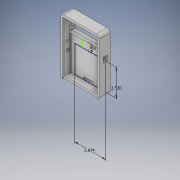
# Autodesk Inventor part: Capstone Calculator
Saved by Autodesk Inventor 2018 (Build 220112000, 112)
## iProperties
Created: 2019-09-20
Part Number: Capstone Calculator
Material: Generic
Document SubType Name: Modeling
Designer: Hyperspin
Density: 1 g/cm^3
Appearance: Default
Author: Hyperspin
Autodesk Inventor part; units mm, degrees
ref_plane "YZ Plane" through (0, 0, 0) normal (1, 0, 0) x (0, 1, 0)
ref_plane "XZ Plane" through (0, 0, 0) normal (0, 1, 0) x (-1, 0, 0)
ref_plane "XY Plane" through (0, 0, 0) normal (0, 0, 1) x (1, 0, 0)
sketch "Sketch1" plane through (0, 0, 0) normal (0, 0, 1) x (1, 0, 0)
  line L0 (0, 0) -> (71, 0)
  line L1 (71, 0) -> (71, 78)
  line L2 (71, 78) -> (0, 78)
  line L3 (0, 78) -> (0, 0)
  line L4 (-4.8, 123.3464) -> (76.2, 123.3464)
  line L5 (76.2, 123.3464) -> (76.2, 86.3464)
  line L6 (76.2, 86.3464) -> (-4.8, 86.3464)
  line L7 (-4.8, 86.3464) -> (-4.8, 123.3464)
  line L8 (-0.5, 90.3464) -> (71.5, 90.3464)
  line L9 (71.5, 90.3464) -> (71.5, 116.3464)
  line L10 (71.5, 116.3464) -> (-0.5, 116.3464)
  line L11 (-0.5, 116.3464) -> (-0.5, 90.3464)
  line L12 (24.5, 0) -> (46.5, 0)
  line L13 (24.5, 0) -> (46.5, 0)
  line L14 (46.5, 0) -> (46.5, 6)
  line L15 (46.5, 6) -> (24.5, 6)
  line L16 (24.5, 6) -> (24.5, 0)
  circle A0 centre (-2.1, 120.6464) radius 1.5
  circle A1 centre (73.5, 120.6464) radius 1.5
  circle A2 centre (-2.1, 89.0464) radius 1.5
  circle A3 centre (73.5, 89.0464) radius 1.5
  dimension "d0" = 71
  dimension "d1" = 78
  dimension "d2" = 37
  dimension "d3" = 81
  dimension "d4" = 72
  dimension "d5" = 26
  dimension "d6" = 4.7
  dimension "d7" = 7
  dimension "d9" = 0.5
  dimension "d14" = 6
  dimension "d15" = 3
  dimension "d16" = 2.7
  dimension "d17" = 2.7
  constraints: 34 end point, 8 parallel, 5 horizontal, 4 centre point, 4 perpendicular, 1 point on line
  measures "d0" distance of L1.end L2.end
  measures "d1" distance of L0.end L1.end
  measures "d2" distance of L4.end L5.end
  measures "d3" distance of L4.start L4.end
  measures "d4" distance of L9.end L10.end
  measures "d5" distance of L8.end L9.end
  measures "d6" distance between parallel lines of L5 L9
  measures "d7" distance between parallel lines of L4 L10
  measures "d9" distance between parallel lines of L3 L11
  measures "d14" distance of L13.end L14.end
  measures "d15" diameter of A0
  measures "d16" distance from line of L4 A0.centre
  measures "d17" distance from line of A0.centre L7
extrude "Extrusion1" add sketch "Sketch1" along normal blind 6.5 contours L3 L2 L1 L0 L14 L15 L16 | L4 L5 L6 L7
sketch "Sketch2" plane through (0, 0, 6.5) normal (0, 0, 1) x (1, 0, 0)
  line L0 (-2.8, 128.3464) -> (74.2, 128.3464)
  line L1 (81.2, 121.3464) -> (81.2, 2)
  line L2 (74.2, -5) -> (-2.8, -5)
  line L3 (-9.8, 2) -> (-9.8, 121.3464)
  line L4 (76.2, 86.3464) -> (76.2, 123.3464) projected
  line L5 (76.2, 123.3464) -> (-4.8, 123.3464) projected
  line L6 (-4.8, 123.3464) -> (-4.8, 86.3464) projected
  line L7 (46.5, 0) -> (71, 0) projected
  arc A0 (-2.8, 128.3464) -> (-9.8, 121.3464) centre (-2.8, 121.3464) ccw
  arc A1 (81.2, 121.3464) -> (74.2, 128.3464) centre (74.2, 121.3464) ccw
  arc A2 (-9.8, 2) -> (-2.8, -5) centre (-2.8, 2) ccw
  arc A3 (74.2, -5) -> (81.2, 2) centre (74.2, 2) ccw
  line L8 (76.2, 123.3464) -> (76.2, 86.3464) projected
  line L9 (-4.8, 123.3464) -> (76.2, 123.3464) projected
  line L10 (-4.8, 86.3464) -> (-4.8, 123.3464) projected
  line L11 (76.2, 86.3464) -> (-4.8, 86.3464) projected
  line L12 (46.5, 0) -> (71, 0) projected
  line L13 (71, 0) -> (0, 0)
  line L14 (0, 0) -> (0, 78)
  line L15 (0, 78) -> (71, 78)
  line L16 (71, 78) -> (71, 0)
  point P0 (0, 0)
  dimension "d20" = 5
  dimension "d21" = 5
  dimension "d22" = 5
  dimension "d23" = 5
  dimension "d24" = 7
  constraints: 16 end point, 8 point on circle, 8 tangent, 4 centre point, 4 parallel, 3 equal radius, 2 horizontal, 2 perpendicular
  measures "d20" distance between parallel lines of L1 L4
  measures "d21" distance between parallel lines of L0 L5
  measures "d22" distance between parallel lines of L3 L6
  measures "d23" distance between parallel lines of L2 L7
  measures "d24" radius of A0
extrude "Extrusion2" add sketch "Sketch2" against normal blind 8.5
sketch "Sketch3" plane through (0, 0, 0) normal (0, 0, -1) x (-1, 0, 0)
  line L0 (-76.2, 86.3464) -> (-76.2, 123.3464) projected
  line L1 (-76.2, 86.3464) -> (4.8, 86.3464) projected
  line L2 (-76.2, 123.3464) -> (4.8, 123.3464)
  line L3 (4.8, 123.3464) -> (4.8, 86.3464)
  line L4 (4.8, 86.3464) -> (-76.2, 86.3464)
  line L5 (-76.2, 86.3464) -> (-76.2, 123.3464)
  line L6 (-71.5, 116.3464) -> (-71.5, 90.3464) projected
  line L7 (0.5, 116.3464) -> (0.5, 90.3464) projected
  line L8 (-71.5, 116.3464) -> (0.5, 116.3464)
  line L9 (0.5, 116.3464) -> (0.5, 90.3464)
  line L10 (0.5, 90.3464) -> (-71.5, 90.3464)
  line L11 (-71.5, 90.3464) -> (-71.5, 116.3464)
  point P0 (0, 0)
  constraints: 16 end point, 4 parallel, 2 horizontal, 2 perpendicular
extrude "Extrusion3" add sketch "Sketch3" along normal up to surface (2 mm away)
sketch "Sketch4" plane through (0, 0, 6.5) normal (0, 0, 1) x (1, 0, 0)
  line L0 (71.5, 116.3464) -> (71.5, 90.3464) projected
  line L1 (-0.5, 116.3464) -> (71.5, 116.3464) projected
  line L2 (71.5, 90.3464) -> (-0.5, 90.3464) projected
  line L3 (0.5, 116.3464) -> (41.5, 116.3464)
  line L4 (-0.5, 90.3464) -> (-0.5, 116.3464) projected
  line L5 (-2.8, 128.3464) -> (74.2, 128.3464) projected
  line L6 (-0.5, 116.3464) -> (-0.5, 90.3464)
  line L7 (-0.5, 96.0971) -> (-5.5585, 96.0971)
  line L8 (-5.5585, 96.0971) -> (-5.5585, 110.5971)
  line L9 (-5.5585, 110.5971) -> (-0.5, 110.5971)
  line L10 (71.5, 116.3464) -> (-0.5, 116.3464)
  line L11 (28.5, 116.3464) -> (28.5, 123.3464)
  line L12 (28.5, 123.3464) -> (70.5, 123.3464)
  line L13 (70.5, 123.3464) -> (70.5, 116.3464)
  line L14 (28.5, 116.3464) -> (70.5, 116.3464)
  line L15 (-0.5, 96.0971) -> (-0.5, 110.5971)
  point P0 (0, 0)
  point P1 (71.5, 96.0971)
  dimension "d37" = 1
  dimension "d38" = 42
  constraints: 22 end point, 4 point on line, 1 collinear, 1 horizontal, 1 vertical
  measures "d37" distance between parallel lines of L13 L0
  measures "d38" distance of L12.start L12.end
extrude "Extrusion4" cut sketch "Sketch4" against normal blind 4
sketch "Sketch5" plane through (0, 0, 6.5) normal (0, 0, 1) x (1, 0, 0)
  line L0 (-4.8, 83.3464) -> (76.2, 83.3464)
  line L1 (76.2, 83.3464) -> (76.2, 0)
  line L2 (76.2, 0) -> (-4.8, 0)
  line L3 (-4.8, 0) -> (-4.8, 83.3464)
  line L4 (-9.8, 2) -> (-9.8, 121.3464) projected
  line L5 (81.2, 121.3464) -> (81.2, 2) projected
  line L6 (71.5, 90.3464) -> (-0.5, 90.3464) projected
  line L7 (46.5, 0) -> (24.5, 0) projected
  point P0 (0, 0)
  dimension "d41" = 5
  dimension "d42" = 5
  dimension "d43" = 7
  dimension "d44" = 0
  constraints: 8 end point, 2 parallel, 1 horizontal, 1 perpendicular
  measures "d41" distance between parallel lines of L3 L4
  measures "d42" distance between parallel lines of L5 L1
  measures "d43" distance between parallel lines of L6 L0
  measures "d44" distance between parallel lines of L7 L2
extrude "Extrusion5" cut sketch "Sketch5" against normal blind 3
sketch "Sketch7" plane through (0, 0, 6.5) normal (0, 0, 1) x (1, 0, 0)
  line L0 (28.5, 116.3464) -> (28.5, 123.3464) projected
  line L1 (28.5, 123.3464) -> (70.5, 123.3464) projected
  line L2 (70.5, 123.3464) -> (70.5, 116.3464) projected
  line L3 (70.5, 116.3464) -> (71.5, 116.3464) projected
  line L4 (71.5, 116.3464) -> (71.5, 90.3464) projected
  line L5 (71.5, 90.3464) -> (-0.5, 90.3464) projected
  line L6 (-0.5, 90.3464) -> (-0.5, 96.0971) projected
  line L7 (-0.5, 96.0971) -> (-5.5585, 96.0971) projected
  line L8 (-5.5585, 96.0971) -> (-5.5585, 110.5971) projected
  line L9 (-5.5585, 110.5971) -> (-0.5, 110.5971) projected
  line L10 (-0.5, 110.5971) -> (-0.5, 116.3464) projected
  line L11 (-0.5, 116.3464) -> (28.5, 116.3464) projected
  line L12 (76.2, 0) -> (-4.8, 0) projected
  line L13 (-4.8, 0) -> (-4.8, 83.3464) projected
  line L14 (-4.8, 83.3464) -> (76.2, 83.3464) projected
  line L15 (76.2, 83.3464) -> (76.2, 0) projected
  line L16 (-2.8, 128.3464) -> (74.2, 128.3464) projected
  arc A0 (-2.8, 128.3464) -> (-9.8, 121.3464) centre (-2.8, 121.3464) ccw projected
  line L17 (-9.8, 2) -> (-9.8, 121.3464) projected
  arc A1 (-9.8, 2) -> (-2.8, -5) centre (-2.8, 2) ccw projected
  line L18 (74.2, -5) -> (-2.8, -5) projected
  arc A2 (74.2, -5) -> (81.2, 2) centre (74.2, 2) ccw projected
  line L19 (81.2, 121.3464) -> (81.2, 2) projected
  arc A3 (81.2, 121.3464) -> (74.2, 128.3464) centre (74.2, 121.3464) ccw projected
  circle A4 centre (73.5, 89.0464) radius 1.5 projected
  circle A5 centre (-2.1, 89.0464) radius 1.5 projected
  circle A6 centre (73.5, 120.6464) radius 1.5 projected
  circle A7 centre (-2.1, 120.6464) radius 1.5 projected
  line L20 (-4.8, 83.3464) -> (76.2, 83.3464)
  line L21 (76.962, 83.3464) -> (76.962, 123.3464)
  line L22 (76.962, 123.3464) -> (-5.5585, 123.3464)
  line L23 (-5.5585, 123.3464) -> (-5.5585, 83.3464)
  line L24 (76.962, 83.3464) -> (76.962, 0)
  line L25 (76.2, 83.3464) -> (76.2, 0) projected
  line L26 (76.962, 0) -> (76.2, 0)
  line L27 (-5.5585, 83.3464) -> (-5.5585, 0)
  line L28 (-5.5585, 0) -> (-4.8, 0)
  point P0 (0, 0)
  dimension "d51" = 0.7585
  dimension "d52" = 0.762
  constraints: 16 end point, 4 perpendicular, 4 point on line, 2 parallel, 1 horizontal, 1 vertical
  measures "d51" distance between parallel lines of L23 L13
  measures "d52" distance between parallel lines of L21 L15
extrude "Extrusion7" add sketch "Sketch7" along normal blind 17 contours L16 A3 L19 A2 L18 A1 L17 A0
sketch "Sketch8" plane through (0, 0, 3.5) normal (0, 0, 1) x (1, 0, 0)
  line L0 (76.2, 83.3464) -> (76.2, 0) projected
  line L1 (76.2, 0) -> (3.2, 0)
  line L2 (3.2, 0) -> (3.2, 64)
  line L3 (3.2, 64) -> (76.2, 64)
  line L4 (76.2, 64) -> (76.2, 0)
  line L5 (33.6587, 64) -> (21.1159, 64)
  line L6 (21.1159, 64) -> (21.1159, 82)
  line L7 (21.1159, 82) -> (33.6587, 82)
  line L8 (33.6587, 82) -> (33.6587, 64)
  point P0 (0, 0)
  dimension "d55" = 73
  dimension "d56" = 64
  dimension "d57" = 18
  constraints: 16 end point, 4 parallel, 2 horizontal, 2 perpendicular, 1 point on line
  measures "d55" distance of L2.end L3.end
  measures "d56" distance between parallel lines of L1 L3
  measures "d57" distance of L7.end L5.start
sketch "Sketch9" plane through (-2.8, -5, -2) normal (0, -1, 0) x (1, 0, 0)
  line L0 (-2.7585, 8.5) -> (-2.7585, 25.5) projected
  line L1 (-2.7585, 21.5) -> (79.762, 21.5)
  line L2 (79.762, 23.5) -> (79.762, 25.5)
  line L3 (79.762, 25.5) -> (-2.7585, 25.5)
  line L4 (-2.7585, 25.5) -> (-2.7585, 23.5)
  line L5 (-2.7585, 21.5) -> (-4.7585, 21.5)
  line L6 (-4.7585, 21.5) -> (-4.7585, 23.5)
  line L7 (-4.7585, 23.5) -> (-2.7585, 23.5)
  line L8 (-2.7585, 23.5) -> (-2.7585, 21.5)
  line L9 (79.762, 25.5) -> (-2.7585, 25.5) projected
  line L10 (79.762, 21.5) -> (81.762, 21.5)
  line L11 (81.762, 21.5) -> (81.762, 23.5)
  line L12 (81.762, 23.5) -> (79.762, 23.5)
  point P0 (2.8, 2)
  dimension "d58" = 4
  dimension "d59" = 2
  dimension "d60" = 2
  constraints: 22 end point, 4 parallel, 2 horizontal, 2 perpendicular, 1 point on line
  measures "d58" distance between parallel lines of L1 L3
  measures "d59" distance of L1.start L5.end
  measures "d60" distance of L5.end L6.end
extrude "Extrusion8" cut sketch "Sketch9" against normal up to surface (128.3464 mm away)
sketch "Sketch10" plane through (-9.8, 2, -2) normal (-1, 0, 0) x (0, 0, 1)
  line L0 (0, 0) -> (0, 119.3464) projected
  line L1 (25.5, -6.4335) -> (25.5, 121.3464) projected
  circle A0 centre (12.75, 77.5) radius 2.9
  line L2 (9.75, 63.5) -> (15.75, 63.5)
  line L3 (15.75, 63.5) -> (15.75, 69.5)
  line L4 (15.75, 69.5) -> (9.75, 69.5)
  line L5 (9.75, 69.5) -> (9.75, 63.5)
  point P0 (2, -2)
  dimension "d63" = 5.8
  dimension "d64" = 6
  dimension "d65" = 6
  dimension "d67" = 8
  dimension "d70" = 63.5
  constraints: 8 end point, 2 parallel, 1 centre point, 1 horizontal, 1 perpendicular
  measures "d63" diameter of A0
  measures "d64" distance of L3.end L4.end
  measures "d65" distance of L2.end L3.end
  measures "d67" distance from line of A0.centre L4
  measures "d70" distance from line of L2 L0.start
extrude "Extrusion9" cut sketch "Sketch10" against normal up to surface (4.2415 mm away)
sketch "Sketch11" plane through (76.962, 0, 6.5) normal (-1, 0, 0) x (0, 0, 1)
  point P0 (-6.5, 0)
sketch "Sketch12" plane through (76.962, 0, 6.5) normal (-1, 0, 0) x (0, 0, 1)
  line L0 (-6.1095, 84.0437) -> (-4.1453, 84.0437)
  line L1 (-4.1453, 84.0437) -> (-4.1453, 62.8671)
  line L2 (-4.1453, 62.8671) -> (-6.1095, 62.8671)
  line L3 (-6.1095, 62.8671) -> (-6.1095, 84.0437)
  line L4 (0, 0) -> (0, 123.3464) projected
  line L5 (0, 77.7054) -> (6, 77.7054)
  line L6 (6, 77.7054) -> (6, 69.2054)
  line L7 (6, 69.2054) -> (0, 69.2054)
  line L8 (0, 69.2054) -> (0, 77.7054)
  line L9 (-6.1095, 73.4554) -> (0, 73.4554)
  line L10 (6, 73.4554) -> (14.2516, 73.4554)
  point P0 (-6.5, 0)
  point P1 (13, 0)
  dimension "d71" = 6
  dimension "d72" = 8.5
  constraints: 20 end point, 4 horizontal, 4 parallel, 3 midpoint, 2 perpendicular, 1 point on line
  measures "d71" distance of L5.start L5.end
  measures "d72" distance of L5.end L6.end
extrude "Extrusion10" cut sketch "Sketch12" against normal up to surface (4.238 mm away) contours L4 L5 L6 L7
sketch "Sketch13" plane through (81.2, 2, -2) normal (1, 0, 0) x (0, 0, -1)
  line L0 (-8.5, 67.2054) -> (-14.5, 67.2054) projected
  line L1 (-14.5, 67.2054) -> (-14.5, 75.7054) projected
  line L2 (-14.5, 75.7054) -> (-8.5, 75.7054) projected
  line L3 (-8.5, 75.7054) -> (-8.5, 67.2054) projected
  line L4 (-16.4563, 77.6617) -> (-16.4563, 65.2491)
  line L5 (-16.4563, 65.2491) -> (-6.5437, 65.2491)
  line L6 (-6.5437, 65.2491) -> (-6.5437, 77.6617)
  line L7 (-6.5437, 77.6617) -> (-16.4563, 77.6617)
  point P0 (-2, -2)
  constraints: 8 end point, 3 other
extrude "Extrusion11" cut sketch "Sketch13" against normal blind 3
sketch "Sketch14" plane through (-5.5585, 0, 6.5) normal (1, 0, 0) x (0, 0, -1)
  line L0 (-1.25, 65.5) -> (-7.25, 65.5) projected
  line L1 (-7.5, 46.0518) -> (-1, 46.0518)
  line L2 (-1, 46.0518) -> (-1, 52.5518)
  line L3 (-1, 52.5518) -> (-7.5, 52.5518)
  line L4 (-7.5, 52.5518) -> (-7.5, 46.0518)
  line L5 (-4.25, 65.5) -> (-4.25, 49.9279)
  point P0 (6.5, 0)
  dimension "d79" = 6.5
  dimension "d80" = 6.5
  dimension "d81" = 3.25
  constraints: 10 end point, 2 parallel, 1 horizontal, 1 midpoint, 1 perpendicular, 1 vertical
  measures "d79" distance of L3.end L1.start
  measures "d80" distance of L1.start L1.end
  measures "d81" distance between parallel lines of L5 L4
extrude "Extrusion12" cut sketch "Sketch14" against normal blind 3
sketch "Sketch15" plane through (-9.8, 2, -2) normal (-1, 0, 0) x (0, 0, 1)
  line L0 (9.5, 50.5518) -> (9.5, 44.0518) projected
  line L1 (9.5, 44.0518) -> (16, 44.0518) projected
  line L2 (9.5, 50.5518) -> (9.5, 44.0518) projected
  line L3 (16, 50.5518) -> (9.5, 50.5518) projected
  line L4 (16, 44.0518) -> (16, 50.5518) projected
  circle A0 centre (12.75, 47.3018) radius 3.25
  line L5 (16, 44.0518) -> (16, 50.5518) projected
  point P0 (2, -2)
  constraints: 1 centre point, 1 tangent
extrude "Extrusion13" cut sketch "Sketch15" against normal up to surface (1.2415 mm away) contours A0
sketch "Sketch16" plane through (-2.8, -5, 19.5) normal (0, 0, 1) x (1, 0, 0)
  line L0 (-2.7585, 0.5665) -> (-2.7585, 128.3464) projected
  line L1 (-2.7585, 128.3464) -> (-2.7585, 5) projected
  arc A0 (-4.7585, 1.8662) -> (0, 0) centre (0, 7) ccw projected
  line L2 (77, 0) -> (0, 0) projected
  line L3 (-2.7585, 5) -> (79.762, 5) projected
  arc A1 (77, 0) -> (81.762, 1.8694) centre (77, 7) ccw projected
  line L4 (-4.7585, 128.3464) -> (-2.7585, 128.3464) projected
  arc A2 (-4.7585, 1.8662) -> (0, 0) centre (0, 7) ccw projected
  line L5 (77, 0) -> (0, 0) projected
  arc A3 (77, 0) -> (81.762, 1.8694) centre (77, 7) ccw projected
  line L6 (81.762, 1.8694) -> (81.762, 128.3464) projected
  line L7 (79.762, 128.3464) -> (81.762, 128.3464) projected
  line L8 (79.762, 5) -> (79.762, 128.3464) projected
  line L9 (-2.7585, 5) -> (79.762, 5) projected
  line L10 (-2.7585, 128.3464) -> (-2.7585, 5) projected
  line L11 (-4.7585, 128.3464) -> (-2.7585, 128.3464) projected
  line L12 (-4.7585, 1.8662) -> (-4.7585, 128.3464) projected
  point P0 (2.8, 5)
extrude "Extrusion14" cut sketch "Sketch16" against normal blind 0.508
body "Solid1"
